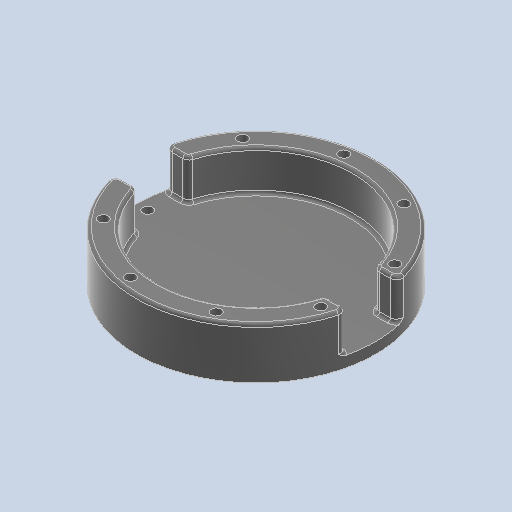
# Autodesk Inventor part: basepart1_forR2
Saved by Autodesk Inventor 2024.3 (Build 283343010, 343A)
## iProperties
Created: 2025-05-25
Part Number: basepart1_forR2
Material: 一般
Document SubType Name: Modeling
Designer: kshau
Density: 1 g/cm^3
Appearance: 滑らか - 黒
Mass: 28.9396 g
Surface Area: 171.356 cm^2
Volume: 28.9396 cm^3
Author: kshau
Autodesk Inventor part; units mm, degrees
ref_plane "YZ Plane" through (0, 0, 0) normal (1, 0, 0) x (0, 1, 0)
ref_plane "XZ Plane" through (0, 0, 0) normal (0, 1, 0) x (-1, 0, 0)
ref_plane "XY Plane" through (0, 0, 0) normal (0, 0, 1) x (1, 0, 0)
sketch "スケッチ1" plane through (0, 0, 0) normal (0, 1, 0) x (-1, 0, 0)
  circle A0 centre (0, 0) radius 40.25
  dimension "d0" = 80.5
  constraints: 1 centre point, 1 coincident
  measures "d0" diameter of A0
extrude "押し出し1" add sketch "スケッチ1" along normal blind 17.2
sketch "スケッチ2" plane through (0, 17.2, 0) normal (0, 1, 0) x (1, 0, 0)
  circle A0 centre (0, 0) radius 32.75
  dimension "d3" = 65.5
  constraints: 1 centre point, 1 coincident
  measures "d3" diameter of A0
extrude "押し出し2" cut sketch "スケッチ2" against normal blind 13.5
sketch "スケッチ3" plane through (0, 17.2, 0) normal (0, 1, 0) x (1, 0, 0)
  circle A0 centre (0, 0) radius 36.5
  point P0 (-36.5, 0)
  point P1 (-27.9606, -23.4617)
  point P2 (-6.3382, -35.9455)
  point P3 (18.25, -31.6099)
  point P4 (34.2988, -12.4837)
  point P5 (34.2988, 12.4837)
  point P6 (18.25, 31.6099)
  point P7 (-6.3382, 35.9455)
  point P8 (-27.9606, 23.4617)
  dimension "d6" = 73
  dimension "d9" = 360
  constraints: 1 coincident, 1 horizontal alignment, 12 other
hole "穴1" at (-36.5, 17.2, 0) at (-27.9606, 17.2, 23.4617) at (-6.3382, 17.2, 35.9455) at (18.25, 17.2, 31.6099) at (34.2988, 17.2, 12.4837) at (34.2988, 17.2, -12.4837) at (18.25, 17.2, -31.6099) at (-6.3382, 17.2, -35.9455) at (-27.9606, 17.2, -23.4617) direction (0, -1, 0) diameter 3.4 end through all
sketch "スケッチ4" plane through (0, 17.2, 0) normal (0, 1, 0) x (1, 0, 0)
  circle A0 centre (0, 0) radius 40.25 projected
  line L0 (39.3458, -8.4837) -> (-39.3458, -8.4837)
  line L1 (0, 0) -> (40.25, 0)
  circle A1 centre (34.2988, -12.4837) radius 1.7 projected
  line L2 (39.3458, 8.4837) -> (-39.3458, 8.4837)
  dimension "d18" = 4
  constraints: 6 end point, 3 point on circle, 2 horizontal, 2 symmetric about line, 1 parallel
  measures "d18" distance from line of A1.centre L0
extrude "押し出し3" cut sketch "スケッチ4" against normal blind 13.5 contours A0 L0 L2
sketch "スケッチ5" plane through (0, 3.7, 0) normal (0, 1, 0) x (1, 0, 0)
  circle A0 centre (-36.5, 0) radius 1.7 projected
  circle A1 centre (-36.5, 0) radius 3
  point P0 (0, 0)
  dimension "d21" = 6
  constraints: 1 centre point, 1 coincident
  measures "d21" diameter of A1
extrude "押し出し4" [suppressed]
sketch "スケッチ6" plane through (0, 0, 0) normal (0, -1, 0) x (1, 0, 0)
  circle A0 centre (-36.5, 0) radius 1.7 projected
  circle A1 centre (-36.5, 0) radius 3
  circle A2 centre (-27.9606, -23.4617) radius 3
  circle A3 centre (-6.3382, -35.9455) radius 3
  circle A4 centre (18.25, -31.6099) radius 3
  circle A5 centre (34.2988, -12.4837) radius 3
  circle A6 centre (34.2988, 12.4837) radius 3
  circle A7 centre (18.25, 31.6099) radius 3
  circle A8 centre (-6.3382, 35.9455) radius 3
  circle A9 centre (-27.9606, 23.4617) radius 3
  point P0 (0, 0)
  dimension "d24" = 6
  dimension "d27" = 360
  constraints: 9 centre point, 1 coincident, 19 other
  measures "d24" diameter of A1
extrude "押し出し5" cut sketch "スケッチ6" against normal blind 3 contours A2 | A3 | A5 | A6 | A8 | A9
fillet "フィレット1" radius 2 8 edges at (31.6321, 10.45, 8.4837) (-31.6321, 10.45, 8.4837) (39.3458, 10.45, 8.4837) (-39.3458, 10.45, 8.4837) (-31.6321, 10.45, -8.4837) (31.6321, 10.45, -8.4837) (-39.3458, 10.45, -8.4837) (39.3458, 10.45, -8.4837)
fillet "フィレット2" radius 1 6 edges at (0, 3.7, 32.75) (-34.958, 3.7, 8.4837) (34.958, 3.7, 8.4837) (0, 3.7, -32.75) (-34.958, 3.7, -8.4837) (34.958, 3.7, -8.4837)
fillet "フィレット3" radius 1 16 edges at (-31.9491, 17.2, 8.8702) (31.9491, 17.2, 8.8702) (-34.958, 17.2, 8.4837) (34.958, 17.2, 8.4837) (38.3815, 17.2, 9.2788) (-38.3815, 17.2, 9.2788) (0, 17.2, 40.25) (0, 17.2, 32.75) (31.9491, 17.2, -8.8702) (-31.9491, 17.2, -8.8702) (34.958, 17.2, -8.4837) (-34.958, 17.2, -8.4837) (38.3815, 17.2, -9.2788) (-38.3815, 17.2, -9.2788) (0, 17.2, -40.25) (0, 17.2, -32.75)
